Autodesk Fusion 360 part; units mm, degrees
(part 2 of 2)
  line L1022 (11.695, 19.049) -> (10.195, 19.049)
  line L1023 (10.195, 19.049) -> (9.445, 17.75)
  line L1024 (9.445, 17.75) -> (10.195, 16.451)
  line L1025 (11.695, 16.451) -> (12.445, 17.75)
  line L1026 (10.195, 16.451) -> (11.695, 16.451)
  line L1027 (15.2725, 16) -> (14.5225, 17.299)
  line L1028 (14.5225, 17.299) -> (13.0225, 17.299)
  line L1029 (13.0225, 17.299) -> (12.2725, 16)
  line L1030 (12.2725, 16) -> (13.0225, 14.701)
  line L1031 (13.0225, 14.701) -> (14.5225, 14.701)
  line L1032 (14.5225, 14.701) -> (15.2725, 16)
  line L1033 (18.0995, 17.75) -> (17.3495, 19.049)
  line L1034 (17.3495, 19.049) -> (15.8495, 19.049)
  line L1035 (15.8495, 19.049) -> (15.0995, 17.75)
  line L1036 (15.0995, 17.75) -> (15.8495, 16.451)
  line L1037 (17.3495, 16.451) -> (18.0995, 17.75)
  line L1038 (15.8495, 16.451) -> (17.3495, 16.451)
  line L1039 (-13, 19.5) -> (-13.75, 20.799)
  line L1040 (-13.75, 20.799) -> (-15.25, 20.799)
  line L1041 (-15.25, 20.799) -> (-16, 19.5)
  line L1042 (-16, 19.5) -> (-15.25, 18.201)
  line L1043 (-15.25, 18.201) -> (-13.75, 18.201)
  line L1044 (-13.75, 18.201) -> (-13, 19.5)
  line L1045 (-10.173, 21.25) -> (-10.923, 22.549)
  line L1046 (-10.923, 22.549) -> (-12.423, 22.549)
  line L1047 (-12.423, 22.549) -> (-13.173, 21.25)
  line L1048 (-13.173, 21.25) -> (-12.423, 19.951)
  line L1049 (-10.923, 19.951) -> (-10.173, 21.25)
  line L1050 (-12.423, 19.951) -> (-10.923, 19.951)
  line L1051 (-7.3455, 19.5) -> (-8.0955, 20.799)
  line L1052 (-8.0955, 20.799) -> (-9.5955, 20.799)
  line L1053 (-9.5955, 20.799) -> (-10.3455, 19.5)
  line L1054 (-10.3455, 19.5) -> (-9.5955, 18.201)
  line L1055 (-9.5955, 18.201) -> (-8.0955, 18.201)
  line L1056 (-8.0955, 18.201) -> (-7.3455, 19.5)
  line L1057 (-4.5185, 21.25) -> (-5.2685, 22.549)
  line L1058 (-5.2685, 22.549) -> (-6.7685, 22.549)
  line L1059 (-6.7685, 22.549) -> (-7.5185, 21.25)
  line L1060 (-7.5185, 21.25) -> (-6.7685, 19.951)
  line L1061 (-5.2685, 19.951) -> (-4.5185, 21.25)
  line L1062 (-6.7685, 19.951) -> (-5.2685, 19.951)
  line L1063 (-1.691, 19.5) -> (-2.441, 20.799)
  line L1064 (-2.441, 20.799) -> (-3.941, 20.799)
  line L1065 (-3.941, 20.799) -> (-4.691, 19.5)
  line L1066 (-4.691, 19.5) -> (-3.941, 18.201)
  line L1067 (-3.941, 18.201) -> (-2.441, 18.201)
  line L1068 (-2.441, 18.201) -> (-1.691, 19.5)
  line L1069 (1.136, 21.25) -> (0.386, 22.549)
  line L1070 (0.386, 22.549) -> (-1.114, 22.549)
  line L1071 (-1.114, 22.549) -> (-1.864, 21.25)
  line L1072 (-1.864, 21.25) -> (-1.114, 19.951)
  line L1073 (0.386, 19.951) -> (1.136, 21.25)
  line L1074 (-1.114, 19.951) -> (0.386, 19.951)
  line L1075 (3.9635, 19.5) -> (3.2135, 20.799)
  line L1076 (3.2135, 20.799) -> (1.7135, 20.799)
  line L1077 (1.7135, 20.799) -> (0.9635, 19.5)
  line L1078 (0.9635, 19.5) -> (1.7135, 18.201)
  line L1079 (1.7135, 18.201) -> (3.2135, 18.201)
  line L1080 (3.2135, 18.201) -> (3.9635, 19.5)
  line L1081 (6.7905, 21.25) -> (6.0405, 22.549)
  line L1082 (6.0405, 22.549) -> (4.5405, 22.549)
  line L1083 (4.5405, 22.549) -> (3.7905, 21.25)
  line L1084 (3.7905, 21.25) -> (4.5405, 19.951)
  line L1085 (6.0405, 19.951) -> (6.7905, 21.25)
  line L1086 (4.5405, 19.951) -> (6.0405, 19.951)
  line L1087 (9.618, 19.5) -> (8.868, 20.799)
  line L1088 (8.868, 20.799) -> (7.368, 20.799)
  line L1089 (7.368, 20.799) -> (6.618, 19.5)
  line L1090 (6.618, 19.5) -> (7.368, 18.201)
  line L1091 (7.368, 18.201) -> (8.868, 18.201)
  line L1092 (8.868, 18.201) -> (9.618, 19.5)
  line L1093 (12.445, 21.25) -> (11.695, 22.549)
  line L1094 (11.695, 22.549) -> (10.195, 22.549)
  line L1095 (10.195, 22.549) -> (9.445, 21.25)
  line L1096 (9.445, 21.25) -> (10.195, 19.951)
  line L1097 (11.695, 19.951) -> (12.445, 21.25)
  line L1098 (10.195, 19.951) -> (11.695, 19.951)
  line L1099 (15.2725, 19.5) -> (14.5225, 20.799)
  line L1100 (14.5225, 20.799) -> (13.0225, 20.799)
  line L1101 (13.0225, 20.799) -> (12.2725, 19.5)
  line L1102 (12.2725, 19.5) -> (13.0225, 18.201)
  line L1103 (13.0225, 18.201) -> (14.5225, 18.201)
  line L1104 (14.5225, 18.201) -> (15.2725, 19.5)
  line L1105 (18.0995, 21.25) -> (17.3495, 22.549)
  line L1106 (17.3495, 22.549) -> (15.8495, 22.549)
  line L1107 (15.8495, 22.549) -> (15.0995, 21.25)
  line L1108 (15.0995, 21.25) -> (15.8495, 19.951)
  line L1109 (17.3495, 19.951) -> (18.0995, 21.25)
  line L1110 (15.8495, 19.951) -> (17.3495, 19.951)
  line L1111 (-13, 23) -> (-13.75, 24.299)
  line L1112 (-13.75, 24.299) -> (-15.25, 24.299)
  line L1113 (-15.25, 24.299) -> (-16, 23)
  line L1114 (-16, 23) -> (-15.25, 21.701)
  line L1115 (-15.25, 21.701) -> (-13.75, 21.701)
  line L1116 (-13.75, 21.701) -> (-13, 23)
  line L1117 (-10.173, 24.75) -> (-10.923, 26.049)
  line L1118 (-10.923, 26.049) -> (-12.423, 26.049)
  line L1119 (-12.423, 26.049) -> (-13.173, 24.75)
  line L1120 (-13.173, 24.75) -> (-12.423, 23.451)
  line L1121 (-10.923, 23.451) -> (-10.173, 24.75)
  line L1122 (-12.423, 23.451) -> (-10.923, 23.451)
  line L1123 (-7.3455, 23) -> (-8.0955, 24.299)
  line L1124 (-8.0955, 24.299) -> (-9.5955, 24.299)
  line L1125 (-9.5955, 24.299) -> (-10.3455, 23)
  line L1126 (-10.3455, 23) -> (-9.5955, 21.701)
  line L1127 (-9.5955, 21.701) -> (-8.0955, 21.701)
  line L1128 (-8.0955, 21.701) -> (-7.3455, 23)
  line L1129 (-4.5185, 24.75) -> (-5.2685, 26.049)
  line L1130 (-5.2685, 26.049) -> (-6.7685, 26.049)
  line L1131 (-6.7685, 26.049) -> (-7.5185, 24.75)
  line L1132 (-7.5185, 24.75) -> (-6.7685, 23.451)
  line L1133 (-5.2685, 23.451) -> (-4.5185, 24.75)
  line L1134 (-6.7685, 23.451) -> (-5.2685, 23.451)
  line L1135 (-1.691, 23) -> (-2.441, 24.299)
  line L1136 (-2.441, 24.299) -> (-3.941, 24.299)
  line L1137 (-3.941, 24.299) -> (-4.691, 23)
  line L1138 (-4.691, 23) -> (-3.941, 21.701)
  line L1139 (-3.941, 21.701) -> (-2.441, 21.701)
  line L1140 (-2.441, 21.701) -> (-1.691, 23)
  line L1141 (1.136, 24.75) -> (0.386, 26.049)
  line L1142 (0.386, 26.049) -> (-1.114, 26.049)
  line L1143 (-1.114, 26.049) -> (-1.864, 24.75)
  line L1144 (-1.864, 24.75) -> (-1.114, 23.451)
  line L1145 (0.386, 23.451) -> (1.136, 24.75)
  line L1146 (-1.114, 23.451) -> (0.386, 23.451)
  line L1147 (3.9635, 23) -> (3.2135, 24.299)
  line L1148 (3.2135, 24.299) -> (1.7135, 24.299)
  line L1149 (1.7135, 24.299) -> (0.9635, 23)
  line L1150 (0.9635, 23) -> (1.7135, 21.701)
  line L1151 (1.7135, 21.701) -> (3.2135, 21.701)
  line L1152 (3.2135, 21.701) -> (3.9635, 23)
  line L1153 (6.7905, 24.75) -> (6.0405, 26.049)
  line L1154 (6.0405, 26.049) -> (4.5405, 26.049)
  line L1155 (4.5405, 26.049) -> (3.7905, 24.75)
  line L1156 (3.7905, 24.75) -> (4.5405, 23.451)
  line L1157 (6.0405, 23.451) -> (6.7905, 24.75)
  line L1158 (4.5405, 23.451) -> (6.0405, 23.451)
  line L1159 (9.618, 23) -> (8.868, 24.299)
  line L1160 (8.868, 24.299) -> (7.368, 24.299)
  line L1161 (7.368, 24.299) -> (6.618, 23)
  line L1162 (6.618, 23) -> (7.368, 21.701)
  line L1163 (7.368, 21.701) -> (8.868, 21.701)
  line L1164 (8.868, 21.701) -> (9.618, 23)
  line L1165 (12.445, 24.75) -> (11.695, 26.049)
  line L1166 (11.695, 26.049) -> (10.195, 26.049)
  line L1167 (10.195, 26.049) -> (9.445, 24.75)
  line L1168 (9.445, 24.75) -> (10.195, 23.451)
  line L1169 (11.695, 23.451) -> (12.445, 24.75)
  line L1170 (10.195, 23.451) -> (11.695, 23.451)
  line L1171 (15.2725, 23) -> (14.5225, 24.299)
  line L1172 (14.5225, 24.299) -> (13.0225, 24.299)
  line L1173 (13.0225, 24.299) -> (12.2725, 23)
  line L1174 (12.2725, 23) -> (13.0225, 21.701)
  line L1175 (13.0225, 21.701) -> (14.5225, 21.701)
  line L1176 (14.5225, 21.701) -> (15.2725, 23)
  line L1177 (18.0995, 24.75) -> (17.3495, 26.049)
  line L1178 (17.3495, 26.049) -> (15.8495, 26.049)
  line L1179 (15.8495, 26.049) -> (15.0995, 24.75)
  line L1180 (15.0995, 24.75) -> (15.8495, 23.451)
  line L1181 (17.3495, 23.451) -> (18.0995, 24.75)
  line L1182 (15.8495, 23.451) -> (17.3495, 23.451)
  line L1183 (-13, 26.5) -> (-13.75, 27.799)
  line L1184 (-13.75, 27.799) -> (-15.25, 27.799)
  line L1185 (-15.25, 27.799) -> (-16, 26.5)
  line L1186 (-16, 26.5) -> (-15.25, 25.201)
  line L1187 (-15.25, 25.201) -> (-13.75, 25.201)
  line L1188 (-13.75, 25.201) -> (-13, 26.5)
  line L1189 (-10.173, 28.25) -> (-10.923, 29.549)
  line L1190 (-10.923, 29.549) -> (-12.423, 29.549)
  line L1191 (-12.423, 29.549) -> (-13.173, 28.25)
  line L1192 (-13.173, 28.25) -> (-12.423, 26.951)
  line L1193 (-10.923, 26.951) -> (-10.173, 28.25)
  line L1194 (-12.423, 26.951) -> (-10.923, 26.951)
  line L1195 (-7.3455, 26.5) -> (-8.0955, 27.799)
  line L1196 (-8.0955, 27.799) -> (-9.5955, 27.799)
  line L1197 (-9.5955, 27.799) -> (-10.3455, 26.5)
  line L1198 (-10.3455, 26.5) -> (-9.5955, 25.201)
  line L1199 (-9.5955, 25.201) -> (-8.0955, 25.201)
  line L1200 (-8.0955, 25.201) -> (-7.3455, 26.5)
  line L1201 (-4.5185, 28.25) -> (-5.2685, 29.549)
  line L1202 (-5.2685, 29.549) -> (-6.7685, 29.549)
  line L1203 (-6.7685, 29.549) -> (-7.5185, 28.25)
  line L1204 (-7.5185, 28.25) -> (-6.7685, 26.951)
  line L1205 (-5.2685, 26.951) -> (-4.5185, 28.25)
  line L1206 (-6.7685, 26.951) -> (-5.2685, 26.951)
  line L1207 (-1.691, 26.5) -> (-2.441, 27.799)
  line L1208 (-2.441, 27.799) -> (-3.941, 27.799)
  line L1209 (-3.941, 27.799) -> (-4.691, 26.5)
  line L1210 (-4.691, 26.5) -> (-3.941, 25.201)
  line L1211 (-3.941, 25.201) -> (-2.441, 25.201)
  line L1212 (-2.441, 25.201) -> (-1.691, 26.5)
  line L1213 (1.136, 28.25) -> (0.386, 29.549)
  line L1214 (0.386, 29.549) -> (-1.114, 29.549)
  line L1215 (-1.114, 29.549) -> (-1.864, 28.25)
  line L1216 (-1.864, 28.25) -> (-1.114, 26.951)
  line L1217 (0.386, 26.951) -> (1.136, 28.25)
  line L1218 (-1.114, 26.951) -> (0.386, 26.951)
  line L1219 (3.9635, 26.5) -> (3.2135, 27.799)
  line L1220 (3.2135, 27.799) -> (1.7135, 27.799)
  line L1221 (1.7135, 27.799) -> (0.9635, 26.5)
  line L1222 (0.9635, 26.5) -> (1.7135, 25.201)
  line L1223 (1.7135, 25.201) -> (3.2135, 25.201)
  line L1224 (3.2135, 25.201) -> (3.9635, 26.5)
  line L1225 (6.7905, 28.25) -> (6.0405, 29.549)
  line L1226 (6.0405, 29.549) -> (4.5405, 29.549)
  line L1227 (4.5405, 29.549) -> (3.7905, 28.25)
  line L1228 (3.7905, 28.25) -> (4.5405, 26.951)
  line L1229 (6.0405, 26.951) -> (6.7905, 28.25)
  line L1230 (4.5405, 26.951) -> (6.0405, 26.951)
  line L1231 (9.618, 26.5) -> (8.868, 27.799)
  line L1232 (8.868, 27.799) -> (7.368, 27.799)
  line L1233 (7.368, 27.799) -> (6.618, 26.5)
  line L1234 (6.618, 26.5) -> (7.368, 25.201)
  line L1235 (7.368, 25.201) -> (8.868, 25.201)
  line L1236 (8.868, 25.201) -> (9.618, 26.5)
  line L1237 (12.445, 28.25) -> (11.695, 29.549)
  line L1238 (11.695, 29.549) -> (10.195, 29.549)
  line L1239 (10.195, 29.549) -> (9.445, 28.25)
  line L1240 (9.445, 28.25) -> (10.195, 26.951)
  line L1241 (11.695, 26.951) -> (12.445, 28.25)
  line L1242 (10.195, 26.951) -> (11.695, 26.951)
  line L1243 (15.2725, 26.5) -> (14.5225, 27.799)
  line L1244 (14.5225, 27.799) -> (13.0225, 27.799)
  line L1245 (13.0225, 27.799) -> (12.2725, 26.5)
  line L1246 (12.2725, 26.5) -> (13.0225, 25.201)
  line L1247 (13.0225, 25.201) -> (14.5225, 25.201)
  line L1248 (14.5225, 25.201) -> (15.2725, 26.5)
  line L1249 (18.0995, 28.25) -> (17.3495, 29.549)
  line L1250 (17.3495, 29.549) -> (15.8495, 29.549)
  line L1251 (15.8495, 29.549) -> (15.0995, 28.25)
  line L1252 (15.0995, 28.25) -> (15.8495, 26.951)
  line L1253 (17.3495, 26.951) -> (18.0995, 28.25)
  line L1254 (15.8495, 26.951) -> (17.3495, 26.951)
  line L1255 (-13, 30) -> (-13.75, 31.299)
  line L1256 (-13.75, 31.299) -> (-15.25, 31.299)
  line L1257 (-15.25, 31.299) -> (-16, 30)
  line L1258 (-16, 30) -> (-15.25, 28.701)
  line L1259 (-15.25, 28.701) -> (-13.75, 28.701)
  line L1260 (-13.75, 28.701) -> (-13, 30)
  line L1261 (-10.173, 31.75) -> (-10.923, 33.049)
  line L1262 (-10.923, 33.049) -> (-12.423, 33.049)
  line L1263 (-12.423, 33.049) -> (-13.173, 31.75)
  line L1264 (-13.173, 31.75) -> (-12.423, 30.451)
  line L1265 (-10.923, 30.451) -> (-10.173, 31.75)
  line L1266 (-12.423, 30.451) -> (-10.923, 30.451)
  line L1267 (-7.3455, 30) -> (-8.0955, 31.299)
  line L1268 (-8.0955, 31.299) -> (-9.5955, 31.299)
  line L1269 (-9.5955, 31.299) -> (-10.3455, 30)
  line L1270 (-10.3455, 30) -> (-9.5955, 28.701)
  line L1271 (-9.5955, 28.701) -> (-8.0955, 28.701)
  line L1272 (-8.0955, 28.701) -> (-7.3455, 30)
  line L1273 (-4.5185, 31.75) -> (-5.2685, 33.049)
  line L1274 (-5.2685, 33.049) -> (-6.7685, 33.049)
  line L1275 (-6.7685, 33.049) -> (-7.5185, 31.75)
  line L1276 (-7.5185, 31.75) -> (-6.7685, 30.451)
  line L1277 (-5.2685, 30.451) -> (-4.5185, 31.75)
  line L1278 (-6.7685, 30.451) -> (-5.2685, 30.451)
  line L1279 (-1.691, 30) -> (-2.441, 31.299)
  line L1280 (-2.441, 31.299) -> (-3.941, 31.299)
  line L1281 (-3.941, 31.299) -> (-4.691, 30)
  line L1282 (-4.691, 30) -> (-3.941, 28.701)
  line L1283 (-3.941, 28.701) -> (-2.441, 28.701)
  line L1284 (-2.441, 28.701) -> (-1.691, 30)
  line L1285 (1.136, 31.75) -> (0.386, 33.049)
  line L1286 (0.386, 33.049) -> (-1.114, 33.049)
  line L1287 (-1.114, 33.049) -> (-1.864, 31.75)
  line L1288 (-1.864, 31.75) -> (-1.114, 30.451)
  line L1289 (0.386, 30.451) -> (1.136, 31.75)
  line L1290 (-1.114, 30.451) -> (0.386, 30.451)
  line L1291 (3.9635, 30) -> (3.2135, 31.299)
  line L1292 (3.2135, 31.299) -> (1.7135, 31.299)
  line L1293 (1.7135, 31.299) -> (0.9635, 30)
  line L1294 (0.9635, 30) -> (1.7135, 28.701)
  line L1295 (1.7135, 28.701) -> (3.2135, 28.701)
  line L1296 (3.2135, 28.701) -> (3.9635, 30)
  line L1297 (6.7905, 31.75) -> (6.0405, 33.049)
  line L1298 (6.0405, 33.049) -> (4.5405, 33.049)
  line L1299 (4.5405, 33.049) -> (3.7905, 31.75)
  line L1300 (3.7905, 31.75) -> (4.5405, 30.451)
  line L1301 (6.0405, 30.451) -> (6.7905, 31.75)
  line L1302 (4.5405, 30.451) -> (6.0405, 30.451)
  line L1303 (9.618, 30) -> (8.868, 31.299)
  line L1304 (8.868, 31.299) -> (7.368, 31.299)
  line L1305 (7.368, 31.299) -> (6.618, 30)
  line L1306 (6.618, 30) -> (7.368, 28.701)
  line L1307 (7.368, 28.701) -> (8.868, 28.701)
  line L1308 (8.868, 28.701) -> (9.618, 30)
  line L1309 (12.445, 31.75) -> (11.695, 33.049)
  line L1310 (11.695, 33.049) -> (10.195, 33.049)
  line L1311 (10.195, 33.049) -> (9.445, 31.75)
  line L1312 (9.445, 31.75) -> (10.195, 30.451)
  line L1313 (11.695, 30.451) -> (12.445, 31.75)
  line L1314 (10.195, 30.451) -> (11.695, 30.451)
  line L1315 (15.2725, 30) -> (14.5225, 31.299)
  line L1316 (14.5225, 31.299) -> (13.0225, 31.299)
  line L1317 (13.0225, 31.299) -> (12.2725, 30)
  line L1318 (12.2725, 30) -> (13.0225, 28.701)
  line L1319 (13.0225, 28.701) -> (14.5225, 28.701)
  line L1320 (14.5225, 28.701) -> (15.2725, 30)
  line L1321 (18.0995, 31.75) -> (17.3495, 33.049)
  line L1322 (17.3495, 33.049) -> (15.8495, 33.049)
  line L1323 (15.8495, 33.049) -> (15.0995, 31.75)
  line L1324 (15.0995, 31.75) -> (15.8495, 30.451)
  line L1325 (17.3495, 30.451) -> (18.0995, 31.75)
  line L1326 (15.8495, 30.451) -> (17.3495, 30.451)
  line L1327 (23.5, 43.9) -> (-28.5, 43.9)
  line L1328 (-28.5, 43.9) -> (-28.5, -43.9)
  line L1329 (-28.5, -43.9) -> (23.5, -43.9)
  line L1330 (23.5, -43.9) -> (23.5, 43.9)
  point P0 (0, 38.5)
  point P1 (0, -39.5)
  point P2 (16.75, 31.75)
  point P3 (-16.75, 31.75)
  point P4 (-16.75, -31.75)
  point P5 (16.75, -31.75)
  point P6 (0, 15)
  point P7 (0, -15)
  point P8 (-14.5, -15)
  point P9 (14.5, -15)
  point P10 (14.5, 15)
  point P11 (-14.5, 15)
  point P12 (-14.5, -29.5)
  point P13 (-11.673, -27.75)
  point P14 (-11.673, -27.75)
  dimension "d10" = 33.5
  dimension "d11" = 63.5
  dimension "d12" = 41
  dimension "d13" = 71
  dimension "d18" = 20.5
  dimension "d20" = 59
  dimension "d21" = 29
  dimension "d22" = 20.5
  dimension "d23" = 1.5
  dimension "d26" = 2.827
  dimension "d27" = 1.75
  dimension "d28" = 1.5
  dimension "d35" = 5.6545
  dimension "d36" = 3.5
  dimension "d58" = 23.5
  dimension "d59" = 28.5
  dimension "d60" = 43.9
  dimension "d61" = 43.9
  dimension "d62" = 52
  dimension "d63" = 3
  constraint coincident L0 origin
  constraint coincident L1 origin
  constraint coincident L2 origin
  constraint coincident L3 origin
  constraint coincident L4 origin
  constraint coincident L5 origin
  constraint coincident L6 P1
  constraint horizontal L7
  constraint perpendicular L7 L8
  constraint parallel L7 L9
  constraint parallel L8 L10
  constraint coincident L11 origin
  constraint coincident L12 origin
  constraint horizontal L13
  constraint perpendicular L13 L14
  constraint parallel L13 L15
  constraint parallel L14 L16
  constraint coincident L17 origin
  constraint coincident L18 origin
  constraint coincident P2 L9.end
  constraint coincident P3 L8.end
  constraint coincident P4 L7.end
  constraint coincident P5 L7.start
  constraint coincident L6 P6
  constraint coincident L20 P6
  constraint coincident L6 P7
  constraint coincident L19 P7
  constraint horizontal L21
  constraint perpendicular L21 L22
  constraint parallel L21 L23
  constraint parallel L22 L24
  constraint coincident L25 origin
  constraint coincident L26 origin
  constraint coincident L19 P8
  constraint coincident L22 P8
  constraint coincident L24 P9
  constraint coincident L19 P9
  constraint coincident L24 P10
  constraint coincident L20 P10
  constraint coincident L22 P11
  constraint coincident L20 P11
  constraint coincident P10 A0.start
  constraint coincident P11 A0.end
  constraint coincident P9 A1.end
  constraint coincident P8 A1.start
  constraint coincident P12 L21.end
  constraint perpendicular L21 L35
  constraint perpendicular L22 L36
  constraint coincident L36 P14
  constraint coincident L35 P14
  constraint coincident P14 P13
  constraint horizontal L1327
  constraint vertical L1328
  constraint horizontal L1329
  constraint vertical L1330
  measures "d10" distance of L8 L10
  measures "d11" distance of L7 L9
  measures "d12" distance of L14 L16
  measures "d13" distance of L13 L15
  measures "d18" distance of L13 L19
  measures "d20" distance of L21 L23
  measures "d21" distance of L22 L24
  measures "d22" distance of L15 L20
  measures "d23" distance of L29.end P12
  measures "d26" distance of P12 L35
  measures "d27" distance of P12 L36
  measures "d28" distance of L37.end P14
  measures "d58" distance of origin L1330
  measures "d59" distance of origin L1328
  measures "d60" distance of origin L1327
  measures "d61" distance of origin L1329
  measures "d62" distance of L1328 L1330
  measures "d63" distance of L16 L1330
extrude "Extrusion3" add sketch "Skizze1" along normal blind 2 contours A0 A1 L27 L28 L49 L50 L51 L53 L55 L56 L57 L67 L68 L69 L73 L74 L75 L76 L77 L109 L110 L113 L115 L116 L117 L120 L151 L152 L153 L154 L155 L157 L158 L159 L160 L236 L237 L238 L247 L248 L252 L308 L309 L310 L311 L319 L320 L323 L324 L380 L381 L382 L383 L391 L392 L395 L396 L452 L453 L454 L455 L463 L464 L467 L468 L524 L525 L526 L527 L535 L536 L539 L540 L596 L597 L598 L599 L607 L608 L611 L612 L668 L669 L670 L671 L679 L680 L683 L684 L740 L741 L742 L743 L751 L752 L755 L756 L812 L813 L814 L815 L823 L824 L827 L828 L884 L885 L886 L887 L895 L896 L899 L900 L956 L957 L958 L959 L967 L968 L971 L972 L1028 L1029 L1030 L1031 L1039 L1043 L1044 L1045 L1046 L1048 L1049 L1050 L1100 L1101 L1102 L1103 L1117 L1121 L1122 L1167 L1168 L1169 L1170 L1195 L1198 L1199 L1200 L1201 L1204 L1205 L1206 L1213 L1215 L1216 L1217 L1218 L1227 L1228 L1229 L1230 L1233 L1234 L1235 L1236 L1282 L1283 L1284 L1294 L1295 L1296
extrude "Extrusion4" add sketch "Skizze1" along normal blind 7 contours L13 L14 L15 L16 | A0 L28 L1027 L1028 L1031 L1032 | A0 L1099 L1100 L1103 L1104 | L28 L955 L956 L959 L960 | A0 L1165 L1166 L1167 L1169 | L28 L883 L884 L887 L888 | A0 L1231 L1232 L1233 L1236 | L28 L811 L812 L815 L816 | A0 L1225 L1226 L1227 L1229 | L28 L739 L740 L743 L744 | A0 L1291 L1292 L1293 L1294 L1296 | L28 L667 L668 L671 L672 | L28 L595 L596 L599 L600 | A0 L1279 L1280 L1281 L1282 L1284 | L28 L523 L524 L527 L528 | A0 L1201 L1202 L1203 L1204 | L28 L451 L452 L455 L456 | A0 L1195 L1196 L1197 L1198 | A1 L28 L379 L380 L383 L384 | A0 L1117 L1118 L1119 L1120 L1122 | A1 L307 L308 L311 L312 | A1 L235 L236 L238 L239 L240 | A0 L1039 L1040 L1041 L1042 L1043 | A1 L157 L160 L161 L162 | A0 L27 L968 L969 L970 L971 | A1 L151 L155 L156 | L27 L896 L897 L898 L899 | A1 L76 L77 L78 | L27 L824 L825 L826 L827 | A1 L67 L69 L70 L71 L72 | L27 L752 L753 L754 L755 | A1 L55 L57 L58 L59 L60 | L27 L680 L681 L682 L683 | A1 L51 L52 L53 L54 | L27 L608 L609 L610 L611 | A1 L117 L118 L119 L120 | L27 L536 L537 L538 L539 | A1 L110 L111 L112 L113 L114 | L27 L464 L465 L466 L467 | A1 L248 L249 L250 L251 L252 | L27 L392 L393 L394 L395 | A1 L27 L320 L321 L322 L323 | L29 L30 L31 L32 L33 L34 | L37 L38 L39 L40 L41 L42 | L43 L44 L45 L46 L47 L48 | L79 L80 L81 L82 L83 L84 | L85 L86 L87 L88 L89 L90 | L91 L92 L93 L94 L95 L96 | L97 L98 L99 L100 L101 L102 | L103 L104 L105 L106 L107 L108 | L163 L164 L165 L166 L167 L168 | L169 L170 L171 L172 L173 L174 | L175 L176 L177 L178 L179 L180 | L241 L242 L243 L244 L245 L246 | L313 L314 L315 L316 L317 L318 | L385 L386 L387 L388 L389 L390 | L457 L458 L459 L460 L461 L462 | L529 L530 L531 L532 L533 L534 | L601 L602 L603 L604 L605 L606 | L673 L674 L675 L676 L677 L678 | L745 L746 L747 L748 L749 L750 | L817 L818 L819 L820 L821 L822 | L889 L890 L891 L892 L893 L894 | L961 L962 L963 L964 L965 L966 | L1033 L1034 L1035 L1036 L1037 L1038 | L1105 L1106 L1107 L1108 L1109 L1110 | L1111 L1112 L1113 L1114 L1115 L1116 | L1171 L1172 L1173 L1174 L1175 L1176 | L1177 L1178 L1179 L1180 L1181 L1182 | L1183 L1184 L1185 L1186 L1187 L1188 | L1189 L1190 L1191 L1192 L1193 L1194 | L1237 L1238 L1239 L1240 L1241 L1242 | L1243 L1244 L1245 L1246 L1247 L1248 | L1249 L1250 L1251 L1252 L1253 L1254 | L1255 L1256 L1257 L1258 L1259 L1260 | L1261 L1262 L1263 L1264 L1265 L1266 | L1267 L1268 L1269 L1270 L1271 L1272 | L1273 L1274 L1275 L1276 L1277 L1278 | L1285 L1286 L1287 L1288 L1289 L1290 | L1297 L1298 L1299 L1300 L1301 L1302 | L1303 L1304 L1305 L1306 L1307 L1308 | L1309 L1310 L1311 L1312 L1313 L1314 | L1315 L1316 L1317 L1318 L1319 L1320 | L1321 L1322 L1323 L1324 L1325 L1326
extrude "Extrusion7" add sketch "Skizze1" along normal blind 2 contours L1327 L1328 L1329 L1330
sketch "Skizze2" plane through (0, 0, 7) normal (0, 0, 1) x (-1, 0, 0)
  arc A0 (14.5, 15) -> (-14.5, 15) centre (0, 15) ccw
  line L0 (14.5, 15) -> (14.5, -15)
  arc A1 (13.124, -21.1652) -> (14.5, -15) centre (0, -15) ccw
  line L1 (13.124, -21.1652) -> (13.173, -21.25)
  line L2 (13.173, -21.25) -> (12.423, -22.549)
  line L3 (12.423, -22.549) -> (12.3799, -22.549)
  arc A2 (1.1696, -29.4528) -> (12.3799, -22.549) centre (0, -15) ccw
  line L4 (1.1696, -29.4528) -> (1.114, -29.549)
  line L5 (1.114, -29.549) -> (-0.386, -29.549)
  line L6 (-0.386, -29.549) -> (-0.4178, -29.494)
  arc A3 (-14.5, -15) -> (-0.4178, -29.494) centre (0, -15) ccw
  line L7 (-14.5, -15) -> (-14.5, 15)
  line L8 (-20.5, -35.5) -> (20.5, -35.5)
  line L9 (20.5, -35.5) -> (20.5, 35.5)
  line L10 (20.5, 35.5) -> (-20.5, 35.5)
  line L11 (-20.5, 35.5) -> (-20.5, -35.5)
  line L12 (-16.75, 31.75) -> (16.75, 31.75) construction
  line L13 (16.75, 31.75) -> (16.75, -31.75) construction
  line L14 (16.75, -31.75) -> (-16.75, -31.75) construction
  line L15 (-16.75, -31.75) -> (-16.75, 31.75) construction
  line L16 (-16.75, 31.75) -> (16.75, -31.75) construction
  line L17 (16.75, 31.75) -> (-16.75, -31.75) construction
  point P0 (16.75, -31.75)
  point P1 (-16.75, -31.75)
  point P2 (-16.75, 31.75)
  point P3 (16.75, 31.75)
  dimension "d43" = 63.5
  dimension "d44" = 33.5
  constraint horizontal L12
  constraint perpendicular L12 L13
  constraint parallel L12 L14
  constraint parallel L13 L15
  constraint coincident L16 origin
  constraint coincident L17 origin
  constraint coincident P0 L13.end
  constraint coincident P1 L14.end
  constraint coincident P2 L12.start
  constraint coincident P3 L12.end
  measures "d43" distance of L12 L14
  measures "d44" distance of L13 L15
hole "Bohrung1" at (-16.75, 31.75, 7) at (16.75, 31.75, 7) at (16.75, -31.75, 7) at (-16.75, -31.75, 7) direction (0, 0, -1) diameter 3.5 depth 6 tip angle 180
ref_plane "Arbeitsebene1" through (0, 0, 2.4) normal (0, 0, 1) x (1, 0, 0)
sketch "Skizze3" plane through (0, 0, 2.4) normal (0, 0, 1) x (1, 0, 0)
  line L0 (16.75, -31.75) -> (-16.75, -31.75) construction
  line L1 (-16.75, -31.75) -> (-16.75, 31.75) construction
  line L2 (-16.75, 31.75) -> (16.75, 31.75) construction
  line L3 (16.75, 31.75) -> (16.75, -31.75) construction
  line L4 (16.75, -31.75) -> (-16.75, 31.75) construction
  line L5 (-16.75, -31.75) -> (16.75, 31.75) construction
  line L6 (18.4532, 28.8) -> (20.1564, 31.75)
  line L7 (20.1564, 31.75) -> (18.4532, 34.7)
  line L8 (18.4532, 34.7) -> (15.0468, 34.7)
  line L9 (15.0468, 34.7) -> (13.3436, 31.75)
  line L10 (13.3436, 31.75) -> (15.0468, 28.8)
  line L11 (15.0468, 28.8) -> (18.4532, 28.8)
  line L12 (-15.0468, 28.8) -> (-13.3436, 31.75)
  line L13 (-13.3436, 31.75) -> (-15.0468, 34.7)
  line L14 (-15.0468, 34.7) -> (-18.4532, 34.7)
  line L15 (-18.4532, 34.7) -> (-20.1564, 31.75)
  line L16 (-20.1564, 31.75) -> (-18.4532, 28.8)
  line L17 (-18.4532, 28.8) -> (-15.0468, 28.8)
  line L18 (-18.4532, -28.8) -> (-20.1564, -31.75)
  line L19 (-20.1564, -31.75) -> (-18.4532, -34.7)
  line L20 (-18.4532, -34.7) -> (-15.0468, -34.7)
  line L21 (-15.0468, -34.7) -> (-13.3436, -31.75)
  line L22 (-13.3436, -31.75) -> (-15.0468, -28.8)
  line L23 (-15.0468, -28.8) -> (-18.4532, -28.8)
  line L24 (15.0468, -28.8) -> (13.3436, -31.75)
  line L25 (13.3436, -31.75) -> (15.0468, -34.7)
  line L26 (15.0468, -34.7) -> (18.4532, -34.7)
  line L27 (18.4532, -34.7) -> (20.1564, -31.75)
  line L28 (20.1564, -31.75) -> (18.4532, -28.8)
  line L29 (18.4532, -28.8) -> (15.0468, -28.8)
  point P0 (16.75, 31.75)
  point P1 (-16.75, 31.75)
  point P2 (-16.75, -31.75)
  point P3 (16.75, -31.75)
  dimension "d49" = 63.5
  dimension "d50" = 33.5
  dimension "d51" = 5.9
  dimension "d52" = 5.9
  dimension "d53" = 5.9
  dimension "d55" = 5.9
  constraint horizontal L0
  constraint perpendicular L0 L1
  constraint parallel L0 L2
  constraint parallel L1 L3
  constraint coincident L4 origin
  constraint coincident L5 origin
  constraint coincident P0 L2.end
  constraint coincident P1 L1.end
  constraint coincident L0.end L1.start
  constraint coincident P3 L0.start
  measures "d49" distance of L0 L2
  measures "d50" distance of L1 L3
  measures "d51" distance of L8 L11
  measures "d52" distance of L14 L17
  measures "d53" distance of L20 L23
  measures "d55" distance of L26 L29
extrude "Extrusion6" cut sketch "Skizze3" along normal blind 2.6
equation "d23 = h"
equation "h = 1.5 mm"
equation "d = 0.5 mm"
equation "d26 = 1.5 * h + 1.154 * d"
equation "d27 = h + d / 2"
equation "d28 = h"
equation "d35 = 3 * h + 2.309 * d"
equation "d36 = 2 * h + d"
